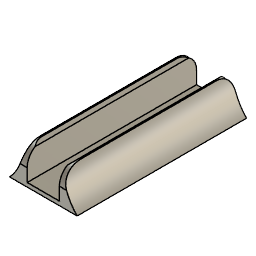
Parametric Notebook Stand (Autodesk Fusion 360 design; units mm, degrees)
Autodesk Fusion 360 part; units mm, degrees
sketch "Sketch1" plane through (0, 0, 0) normal (0, 1, 0) x (1, 0, 0)
  line L0 (0, 0) -> (0, -10) construction
  line L1 (-4.75, -10) -> (4.75, -10) construction
  line L2 (4.75, -10) -> (4.75, -1.2)
  line L3 (-4.75, -10) -> (-4.75, -1.2)
  line L4 (-4.75, -1.2) -> (4.75, -1.2)
  line L5 (-5.95, -10) -> (-5.95, 0) construction
  line L6 (-5.95, 0) -> (5.95, 0)
  line L7 (5.95, -10) -> (5.95, 0) construction
  line L8 (-10, 0) -> (10, 0)
  line L9 (-4.75, -10) -> (-5.95, -10)
  line L10 (4.75, -10) -> (5.95, -10)
  arc A0 (10, 0) -> (5.95, -10) centre (20.3207, -10) ccw
  arc A1 (-5.95, -10) -> (-10, 0) centre (-20.3207, -10) ccw
  dimension "d1" = 9.5
  dimension "d5" = -1.2
  dimension "d6" = 20
  dimension "d15" = 10
  constraint coincident L0.start origin
  constraint vertical L0
  constraint horizontal L1
  constraint midpoint L0.end L1
  constraint perpendicular L2 L4
  constraint horizontal L8
  constraint midpoint L8 L0.start
  constraint vertical L0.start origin
  constraint collinear L6 L8
  constraint tangent L7 A0
  constraint vertical L3
  constraint tangent L5 A1
  constraint equal A0 A1
  constraint horizontal L9
  measures "d1" distance of L1.start L1.end
  measures "d6" distance of L8.start L8.end
  measures "d15" distance of L0.start L0.end
extrude "Extrude1" add sketch "Sketch1" along normal blind 50
chamfer "Chamfer2" distance 0.8 angle 45 2 edges at (4.75, 25, 10) (-4.75, 25, 10)
fillet "Fillet1" radius 5 4 edges at (-5.75, 0, 10) (5.75, 0, 10) (5.75, 50, 10) (-5.75, 50, 10)
equation "d1 = thickness"
equation "d6 = thickness + 10.5 mm"
equation "d7 = width"
equation "thickness = 9.5 mm"
equation "height = 10 mm"
equation "d15 = height"
equation "width = 50 mm"
